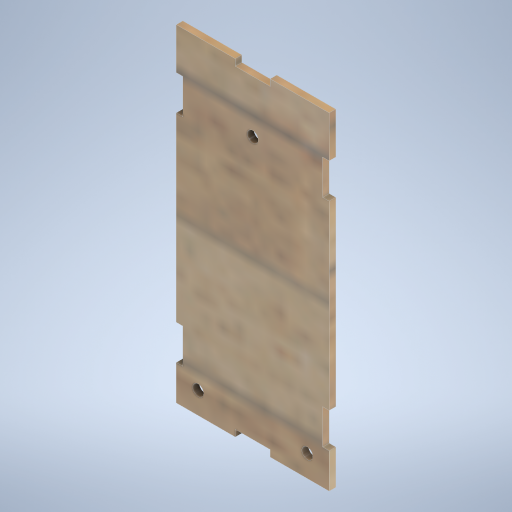
# Autodesk Inventor part: bottom plate
Saved by Autodesk Inventor 2023 (Build 270158000, 158)
## iProperties
Created: 2023-06-06
Part Number: bottom plate
Material: Hardboard
Document SubType Name: Sheet Metal
Designer: Ronan
Density: 0.799949 g/cm^3
Sheet Metal Rule: Default_mm
Appearance: Natural Maple - Glossy Dark Tint(1)
Author: Ronan
Autodesk Inventor part; units mm, degrees
ref_plane "YZ Plane" through (0, 0, 0) normal (1, 0, 0) x (0, 1, 0)
ref_plane "XZ Plane" through (0, 0, 0) normal (0, 1, 0) x (-1, 0, 0)
ref_plane "XY Plane" through (0, 0, 0) normal (0, 0, 1) x (1, 0, 0)
sketch "Sketch1" plane through (0, 0, 0) normal (0, 0, 1) x (1, 0, 0)
  line L0 (0, 0) -> (70, 0)
  line L1 (70, 0) -> (70, 150)
  line L2 (0, 131) -> (3, 131)
  line L3 (3, 131) -> (3, 115)
  line L4 (3, 115) -> (0, 115)
  line L5 (0, 115) -> (0, 131)
  line L6 (0, 32) -> (3, 32)
  line L7 (3, 32) -> (3, 16)
  line L8 (3, 16) -> (0, 16)
  line L9 (0, 16) -> (0, 32)
  line L10 (70, 131) -> (67, 131)
  line L11 (67, 131) -> (67, 115)
  line L12 (67, 115) -> (70, 115)
  line L13 (70, 115) -> (70, 131)
  line L14 (70, 32) -> (67, 32)
  line L15 (67, 32) -> (67, 16)
  line L16 (67, 16) -> (70, 16)
  line L17 (70, 16) -> (70, 32)
  line L18 (43, 150) -> (43, 147)
  line L19 (43, 147) -> (27, 147)
  line L20 (27, 147) -> (27, 150)
  line L21 (70, 150) -> (43, 150)
  line L22 (27, 150) -> (0, 150)
  line L23 (0, 150) -> (0, 131)
  line L24 (0, 115) -> (0, 0)
  line L25 (43, 0) -> (27, 0)
  line L26 (27, 0) -> (27, 3)
  line L27 (27, 3) -> (43, 3)
  line L28 (43, 3) -> (43, 0)
  point P0 (1.5, 16)
  point P1 (70, 123)
  point P2 (67, 123)
  dimension "d1" = 70
  dimension "d2" = 16
  dimension "d3" = 16
  dimension "d4" = 16
  dimension "d9" = 16
  dimension "d12" = 19
  dimension "d13" = 150
  dimension "d15" = 3
  dimension "d16" = 3
  dimension "d17" = 3
  measures "d1" distance of L1.end L22.end
  measures "d2" distance of L2.end L3.end
  measures "d3" distance of L6.end L7.end
  measures "d4" distance from line of point (1.5, 16) L0
  measures "d9" distance of L18.end L19.end
  measures "d12" distance between parallel lines of L22 L2
  measures "d13" distance of L22.end L0.start
  measures "d15" distance of L2.start L2.end
  measures "d16" distance of L10.start L10.end
  measures "d17" distance of L19.end L20.end
extrude "Plate1" add sketch "Sketch1" along normal blind 3 contours L24 L8 L7 L6 L4 L3 L2 L23 L22 L20 L19 L18 L21 L1 L10 L11 L12 L14 L15 L16 L0 L28 L27 L26
sketch "Sketch2" plane through (0, 0, 0) normal (0, 0, -1) x (-1, 0, 0)
  circle A0 centre (-35, 123) radius 2.5
  circle A1 centre (-60, 10) radius 2.5
  circle A2 centre (-10, 10) radius 2.5
  line L0 (-43, 147) -> (-27, 147) projected
  line L1 (-67, 131) -> (-67, 115) projected
  line L2 (-3, 131) -> (-3, 115) projected
  line L3 (0, 16) -> (-3, 16) projected
  line L4 (0, 0) -> (-27, 0) projected
  line L5 (0, 16) -> (0, 0) projected
  line L6 (-70, 0) -> (-70, 16) projected
  point P0 (-1.5, 16)
  point P1 (0, 8)
  dimension "d18" = 24
  dimension "d19" = 32
  dimension "d20" = 32
  dimension "d21" = 5
  dimension "d23" = 5
  dimension "d24" = 10
  dimension "d25" = 10
  dimension "d26" = 10
  constraints: 3 centre point, 2 midpoint, 1 equal radius, 1 horizontal alignment
  measures "d18" distance from line of L0 A0.centre
  measures "d19" distance from line of A0.centre L1
  measures "d20" distance from line of L2 A0.centre
  measures "d21" diameter of A0
  measures "d23" diameter of A2
  measures "d24" distance from line of L4 A2.centre
  measures "d25" horizontal distance of point (0, 8) A2.centre
  measures "d26" distance from line of L6 A1.centre
extrude "Extrusion1" cut sketch "Sketch2" against normal through all
equation "\"d14\" = Thickness"
equation "\"BendRadius\" = Thickness"
equation "\"BendReliefWidth\" = Thickness"
equation "\"BendReliefDepth\" = 0.5 * Thickness"
equation "\"CornerReliefSize\" = 4 * Thickness"
equation "\"MinimumRemnant\" = 2 * Thickness"
equation "\"TransitionRadius\" = BendRadius"
equation "\"JacobiRadiusSize\" = BendRadius"
equation "\"GapSize\" = Thickness"
equation "\"Thickness\" = 3"
body "Solid1"
